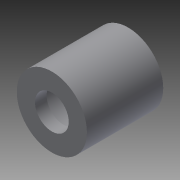
# Autodesk Inventor part: Magnet to Igus adapter
Saved by Autodesk Inventor 2014 (Build 180170000, 170)
## iProperties
Created: 2014-02-09
Part Number: Magnet to Igus adapter
Material: Generic
Document SubType Name: Modeling
Designer: Spooner
Density: 1 g/cm^3
Appearance: Default
Author: Spooner
Autodesk Inventor part; units mm, degrees
ref_plane "YZ Plane" through (0, 0, 0) normal (1, 0, 0) x (0, 1, 0)
ref_plane "XZ Plane" through (0, 0, 0) normal (0, 1, 0) x (-1, 0, 0)
ref_plane "XY Plane" through (0, 0, 0) normal (0, 0, 1) x (1, 0, 0)
sketch "Sketch1" plane through (0, 0, 0) normal (0, 0, 1) x (1, 0, 0)
  circle A0 centre (0, 0) radius 8.0328
  circle A1 centre (0, 0) radius 10.5727
  dimension "d0" = 16.0655
  dimension "d3" = 2.54
  constraints: 2 centre point, 2 coincident
  measures "d0" diameter of A0
  measures "d3" radial gap between concentric circles of A1 A0
extrude "Extrusion1" add sketch "Sketch1" along normal blind 6.35
sketch "Sketch3" plane through (0, 0, 6.35) normal (0, 0, 1) x (1, 0, 0)
  circle A0 centre (0, 0) radius 10.5727 projected
  circle A1 centre (0, 0) radius 10.5727
  circle A2 centre (0, 0) radius 8.0328
  circle A3 centre (0, 0) radius 8.0328 projected
  constraints: 2 centre point, 2 coincident, 2 concentric
extrude "Extrusion2" add sketch "Sketch3" along normal blind 6.2738
sketch "Sketch7" plane through (0, 0, 12.6238) normal (0, 0, 1) x (1, 0, 0)
  circle A0 centre (0, 0) radius 10.5727 projected
  circle A1 centre (0, 0) radius 7.5882
  dimension "d12" = 15.1765
  constraints: 1 centre point, 1 coincident
  measures "d12" diameter of A1
extrude "Extrusion4" add sketch "Sketch7" along normal blind 6.858
sketch "Sketch8" plane through (0, 0, 19.4818) normal (0, 0, 1) x (1, 0, 0)
  circle A0 centre (0, 0) radius 10.5727 projected
  circle A1 centre (0, 0) radius 5.0864
  dimension "d15" = 10.1727
  constraints: 1 centre point, 1 coincident
  measures "d15" diameter of A1
extrude "Extrusion5" add sketch "Sketch8" along normal blind 3.5179
body "Solid1"
